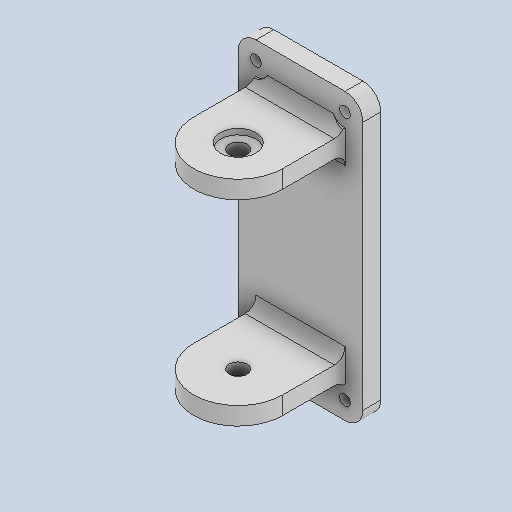
# Autodesk Inventor part: UnionBrazoPantalla
Saved by Autodesk Inventor 2023 (Build 270158000, 158)
## iProperties
Created: 2023-05-13
Part Number: UnionBrazoPantalla
Material: Genérico
Document SubType Name: Modeling
Designer: sergi
Density: 1 g/cm^3
Appearance: Valor por defecto
Author: sergi
Autodesk Inventor part; units mm, degrees
note: some values were not read from the file. Chosen so that the rebuilt part matches the saved one: direction of "Agujero1"; direction of "Agujero2".
ref_plane "YZ Plane" through (0, 0, 0) normal (1, 0, 0) x (0, 1, 0)
ref_plane "XZ Plane" through (0, 0, 0) normal (0, 1, 0) x (-1, 0, 0)
ref_plane "XY Plane" through (0, 0, 0) normal (0, 0, 1) x (1, 0, 0)
sketch "Boceto1" plane through (0, 0, 0) normal (0, 0, 1) x (1, 0, 0)
  line L0 (75.85, 9) -> (75.85, -9) projected
  line L1 (75.85, 9) -> (95.85, 9) projected
  line L2 (95.85, -9) -> (95.85, 9) projected
  line L3 (105.85, -146.9) -> (105.85, 146.9) projected
  line L4 (105.85, 146.9) -> (112.15, 146.9) projected
  line L5 (112.15, 146.9) -> (112.15, 160) projected
  line L6 (112.15, 160) -> (105.85, 160) projected
  line L7 (105.85, 160) -> (105.85, 180) projected
  line L8 (105.85, 180) -> (-100.9, 180) projected
  line L9 (-100.9, 180) -> (-100.9, 160) projected
  line L10 (-100.9, 160) -> (-108.4, 160) projected
  line L11 (-108.4, 160) -> (-108.4, 145) projected
  line L12 (-108.4, 145) -> (-100.9, 145) projected
  line L13 (-100.9, 145) -> (-100.9, 142) projected
  line L14 (-100.9, 142) -> (-112.15, 142) projected
  line L15 (-112.15, 142) -> (-112.15, -142) projected
  line L16 (15.85, 9) -> (15.85, -9) projected
  line L17 (15.85, 9) -> (35.85, 9) projected
  line L18 (35.85, -9) -> (35.85, 9) projected
  line L19 (20.45, 169.8) -> (20.45, 163.3) projected
  line L20 (20.45, 163.3) -> (13.95, 163.3) projected
  line L21 (13.95, 163.3) -> (13.95, 169.8) projected
  line L22 (13.95, 169.8) -> (20.45, 169.8) projected
  line L23 (78.15, 169.8) -> (78.15, 163.3) projected
  line L24 (78.15, 163.3) -> (71.65, 163.3) projected
  line L25 (71.65, 163.3) -> (71.65, 169.8) projected
  line L26 (71.65, 169.8) -> (78.15, 169.8) projected
  line L27 (-4.15, 163.3) -> (-4.15, 169.8) projected
  line L28 (-4.15, 169.8) -> (2.35, 169.8) projected
  line L29 (2.35, 169.8) -> (2.35, 163.3) projected
  line L30 (2.35, 163.3) -> (-4.15, 163.3) projected
  line L31 (38.55, 169.8) -> (38.55, 163.3) projected
  line L32 (38.55, 163.3) -> (32.05, 163.3) projected
  line L33 (32.05, 163.3) -> (32.05, 169.8) projected
  line L34 (32.05, 169.8) -> (38.55, 169.8) projected
  line L35 (56.65, 169.8) -> (56.65, 163.3) projected
  line L36 (56.65, 163.3) -> (50.15, 163.3) projected
  line L37 (50.15, 163.3) -> (50.15, 169.8) projected
  line L38 (50.15, 169.8) -> (56.65, 169.8) projected
  line L39 (-14.65, 175.8) -> (-14.65, 157.7) projected
  line L40 (-14.65, 157.7) -> (-22.65, 157.7) projected
  line L41 (-22.65, 157.7) -> (-22.65, 175.8) projected
  line L42 (-22.65, 175.8) -> (-14.65, 175.8) projected
  line L43 (35.85, -9) -> (35.85, 9) projected
  line L44 (35.85, -9) -> (15.85, -9) projected
  line L45 (15.85, 9) -> (15.85, -9) projected
  line L46 (-112.15, 142) -> (-112.15, -142) projected
  line L47 (-112.15, -142) -> (-100.9, -142) projected
  line L48 (-100.9, -142) -> (-100.9, -145) projected
  line L49 (-100.9, -145) -> (-108.4, -145) projected
  line L50 (-108.4, -145) -> (-108.4, -160) projected
  line L51 (-108.4, -160) -> (-100.9, -160) projected
  line L52 (-100.9, -160) -> (-100.9, -180) projected
  line L53 (-100.9, -180) -> (105.85, -180) projected
  line L54 (105.85, -180) -> (105.85, -160) projected
  line L55 (105.85, -160) -> (112.15, -160) projected
  line L56 (112.15, -160) -> (112.15, -146.9) projected
  line L57 (112.15, -146.9) -> (105.85, -146.9) projected
  line L58 (105.85, -146.9) -> (105.85, 146.9) projected
  line L59 (95.85, -9) -> (95.85, 9) projected
  line L60 (95.85, -9) -> (75.85, -9) projected
  line L61 (75.85, 9) -> (75.85, -9) projected
  circle A0 centre (-103.8, -156.7) radius 1.5 projected
  line L62 (-25.85, -52.4) -> (-25.85, -57.4) projected
  line L63 (-25.85, -57.4) -> (-8.15, -57.4) projected
  arc A1 (-3.15, -62.4) -> (-8.15, -57.4) centre (-8.15, -62.4) ccw projected
  line L64 (-3.15, -62.4) -> (-3.15, -87.4) projected
  line L65 (-3.15, -87.4) -> (-2.05, -87.4) projected
  line L66 (-2.05, -87.4) -> (-2.05, -107.4) projected
  line L67 (-2.05, -107.4) -> (-3.15, -107.4) projected
  line L68 (-3.15, -107.4) -> (-3.15, -169.7804) projected
  arc A2 (-8.15, -174.7804) -> (-3.15, -169.7804) centre (-8.15, -169.7804) ccw projected
  line L69 (-8.15, -174.7804) -> (-67.5256, -174.7804) projected
  line L70 (-67.5256, -174.7804) -> (-67.5256, -57.4) projected
  line L71 (-67.5256, -57.4) -> (-48.05, -57.4) projected
  line L72 (-48.05, -57.4) -> (-48.05, -52.4) projected
  line L73 (-48.05, -52.4) -> (-25.85, -52.4) projected
  line L74 (-112.15, 0) -> (-67.15, 0)
  line L75 (-67.15, 0) -> (-67.15, -40)
  line L76 (-67.15, -40) -> (-32.15, -40)
  line L77 (-32.15, -40) -> (-32.15, 40)
  line L78 (-32.15, 40) -> (-67.15, 40)
  line L79 (-67.15, 40) -> (-67.15, 0)
  line L80 (-37.15, 35) -> (-37.15, -35)
  line L81 (-37.15, -35) -> (-62.15, -35)
  line L82 (-62.15, -35) -> (-62.15, 0)
  line L83 (-62.15, 0) -> (-62.15, 35)
  line L84 (-62.15, 35) -> (-37.15, 35)
  circle A3 centre (-37.15, 35) radius 1.5
  circle A4 centre (-37.15, -35) radius 1.5
  circle A5 centre (-62.15, -35) radius 1.5
  circle A6 centre (-62.15, 35) radius 1.5
  circle A7 centre (-37.15, -35) radius 1.6 projected
  circle A8 centre (-37.15, 35) radius 1.6 projected
  circle A9 centre (-62.15, 35) radius 1.6 projected
  circle A10 centre (-62.15, -35) radius 1.6 projected
  line L85 (75.85, 9) -> (95.85, 9) projected
  line L86 (15.85, 9) -> (35.85, 9) projected
  line L87 (20.45, 169.8) -> (20.45, 163.3) projected
  line L88 (20.45, 163.3) -> (13.95, 163.3) projected
  line L89 (13.95, 163.3) -> (13.95, 169.8) projected
  line L90 (13.95, 169.8) -> (20.45, 169.8) projected
  line L91 (78.15, 169.8) -> (78.15, 163.3) projected
  line L92 (78.15, 163.3) -> (71.65, 163.3) projected
  line L93 (71.65, 163.3) -> (71.65, 169.8) projected
  line L94 (71.65, 169.8) -> (78.15, 169.8) projected
  line L95 (-4.15, 163.3) -> (-4.15, 169.8) projected
  line L96 (-4.15, 169.8) -> (2.35, 169.8) projected
  line L97 (2.35, 169.8) -> (2.35, 163.3) projected
  line L98 (2.35, 163.3) -> (-4.15, 163.3) projected
  line L99 (38.55, 169.8) -> (38.55, 163.3) projected
  line L100 (38.55, 163.3) -> (32.05, 163.3) projected
  line L101 (32.05, 163.3) -> (32.05, 169.8) projected
  line L102 (32.05, 169.8) -> (38.55, 169.8) projected
  line L103 (56.65, 169.8) -> (56.65, 163.3) projected
  line L104 (56.65, 163.3) -> (50.15, 163.3) projected
  line L105 (50.15, 163.3) -> (50.15, 169.8) projected
  line L106 (50.15, 169.8) -> (56.65, 169.8) projected
  line L107 (-14.65, 175.8) -> (-14.65, 157.7) projected
  line L108 (-14.65, 157.7) -> (-22.65, 157.7) projected
  line L109 (-22.65, 157.7) -> (-22.65, 175.8) projected
  line L110 (-22.65, 175.8) -> (-14.65, 175.8) projected
  line L111 (-100.9, 142) -> (-112.15, 142) projected
  line L112 (105.85, 146.9) -> (112.15, 146.9) projected
  line L113 (112.15, 146.9) -> (112.15, 160) projected
  line L114 (112.15, 160) -> (105.85, 160) projected
  line L115 (105.85, 160) -> (105.85, 180) projected
  line L116 (105.85, 180) -> (-100.9, 180) projected
  line L117 (-100.9, 180) -> (-100.9, 160) projected
  line L118 (-100.9, 160) -> (-108.4, 160) projected
  line L119 (-108.4, 160) -> (-108.4, 145) projected
  line L120 (-108.4, 145) -> (-100.9, 145) projected
  line L121 (-100.9, 145) -> (-100.9, 142) projected
  circle A11 centre (-37.15, -35) radius 1.6 projected
  circle A12 centre (-37.15, 35) radius 1.6 projected
  circle A13 centre (-62.15, 35) radius 1.6 projected
  circle A14 centre (-62.15, -35) radius 1.6 projected
  line L122 (95.85, -9) -> (75.85, -9) projected
  line L123 (35.85, -9) -> (15.85, -9) projected
  line L124 (-25.85, -52.4) -> (-25.85, -57.4) projected
  line L125 (-25.85, -57.4) -> (-8.15, -57.4) projected
  arc A15 (-3.15, -62.4) -> (-8.15, -57.4) centre (-8.15, -62.4) ccw projected
  line L126 (-3.15, -62.4) -> (-3.15, -87.4) projected
  line L127 (-3.15, -87.4) -> (-2.05, -87.4) projected
  line L128 (-2.05, -87.4) -> (-2.05, -107.4) projected
  line L129 (-2.05, -107.4) -> (-3.15, -107.4) projected
  line L130 (-3.15, -107.4) -> (-3.15, -169.7804) projected
  arc A16 (-8.15, -174.7804) -> (-3.15, -169.7804) centre (-8.15, -169.7804) ccw projected
  line L131 (-8.15, -174.7804) -> (-67.5256, -174.7804) projected
  line L132 (-67.5256, -174.7804) -> (-67.5256, -57.4) projected
  line L133 (-67.5256, -57.4) -> (-48.05, -57.4) projected
  line L134 (-48.05, -57.4) -> (-48.05, -52.4) projected
  line L135 (-48.05, -52.4) -> (-25.85, -52.4) projected
  circle A17 centre (-103.8, -156.7) radius 1.5 projected
  line L136 (-112.15, -142) -> (-100.9, -142) projected
  line L137 (-100.9, -142) -> (-100.9, -145) projected
  line L138 (-100.9, -145) -> (-108.4, -145) projected
  line L139 (-108.4, -145) -> (-108.4, -160) projected
  line L140 (-108.4, -160) -> (-100.9, -160) projected
  line L141 (-100.9, -160) -> (-100.9, -180) projected
  line L142 (-100.9, -180) -> (105.85, -180) projected
  line L143 (105.85, -180) -> (105.85, -160) projected
  line L144 (105.85, -160) -> (112.15, -160) projected
  line L145 (112.15, -160) -> (112.15, -146.9) projected
  line L146 (112.15, -146.9) -> (105.85, -146.9) projected
  dimension "d0" = 45
  dimension "d1" = 40
  dimension "d2" = 35
  dimension "d3" = 80
  dimension "d4" = 5
  dimension "d5" = 3
  dimension "d6" = 3
  dimension "d7" = 3
  dimension "d8" = 3
  constraints: 22 end point, 8 perpendicular, 4 centre point, 4 coincident, 1 point on line, 4 other
  measures "d0" distance of L74.start L74.end
  measures "d1" distance of L74.end L75.end
  measures "d2" distance of L75.end L76.end
  measures "d3" distance of L76.end L77.end
  measures "d4" distance between parallel lines of L77 L80
  measures "d5" diameter of A3
  measures "d6" diameter of A4
  measures "d7" diameter of A5
  measures "d8" diameter of A6
extrude "Extrusión1" add sketch "Boceto1" along normal blind 5 contours L79 L78 L77 L76 L75 | A3 L84 A8 L80 | L80 A8 L84 A3 | L80 A7 L81 A10 L82 L83 A9 L84 A8 | A7 L81 A4 L80 | L80 A4 L81 A7 | A9 L83 A6 L84 | L84 A6 L83 A9 | A10 L82 A5 L81 | L81 A5 L82 A10
sketch "Boceto2" plane through (0, 0, 5) normal (0, 0, 1) x (1, 0, 0)
  circle A0 centre (-37.15, 35) radius 1.5 projected
  circle A1 centre (-62.15, -35) radius 1.5 projected
  line L0 (-37.15, 35) -> (-62.15, 35)
  line L1 (-62.15, 35) -> (-62.15, -35)
  line L2 (-62.15, -35) -> (-37.15, -35)
  line L3 (-37.15, -35) -> (-37.15, 35)
  line L4 (-50.6099, 35) -> (-50.6099, 30)
  line L5 (-37.15, 30) -> (-62.15, 30)
  line L6 (-37.15, 25) -> (-62.15, 25)
  line L7 (-49.65, -35) -> (-49.65, -30)
  line L8 (-49.65, -25) -> (-37.15, -25)
  line L9 (-49.65, -30) -> (-37.15, -30)
  line L10 (-49.65, -30) -> (-62.15, -30)
  line L11 (-62.15, -30) -> (-37.15, -30)
  line L12 (-37.15, -30) -> (-37.15, -25)
  line L13 (-37.15, -25) -> (-62.15, -25)
  line L14 (-62.15, -25) -> (-62.15, -30)
  point P0 (0, 0)
  dimension "d11" = 5
  dimension "d12" = 5
  dimension "d13" = 5
  dimension "d14" = 5
  constraints: 30 end point, 8 point on line, 6 parallel, 4 perpendicular, 3 horizontal, 1 midpoint, 1 vertical
  measures "d11" distance of L4.start L4.end
  measures "d12" distance between parallel lines of L5 L6
  measures "d13" distance of L7.start L7.end
  measures "d14" distance of L7.end L8.start
extrude "Extrusión2" add sketch "Boceto2" along normal blind 30 contours L3 L6 L1 L5 | L3 L9 L10 L1 L13 L8
fillet "Empalme1" radius 12.5 4 edges at (-37.15, 27.5, 35) (-62.15, 27.5, 35) (-37.15, -27.5, 35) (-62.15, -27.5, 35)
fillet "Empalme2" radius 3 4 edges at (-49.65, 30, 5) (-49.65, 25, 5) (-49.65, -25, 5) (-49.65, -30, 5)
sketch "Boceto3" plane through (0, 0, 5) normal (0, 0, 1) x (1, 0, 0)
  line L0 (-62.15, -33) -> (-62.15, -22) projected
  line L1 (-37.15, -22) -> (-62.15, -22) projected
  line L2 (-37.15, -22) -> (-37.15, -33) projected
  line L3 (-62.15, -33) -> (-37.15, -33) projected
  line L4 (-62.15, 22) -> (-62.15, 33) projected
  line L5 (-37.15, 33) -> (-62.15, 33) projected
  line L6 (-37.15, 33) -> (-37.15, 22) projected
  line L7 (-62.15, 22) -> (-37.15, 22) projected
  line L8 (-32.15, 40) -> (-67.15, 40) projected
  line L9 (-67.15, 40) -> (-67.15, -40) projected
  line L10 (-67.15, -40) -> (-32.15, -40) projected
  line L11 (-32.15, -40) -> (-32.15, 40) projected
  circle A0 centre (-62.15, -35) radius 1.5 projected
  circle A1 centre (-37.15, -35) radius 1.5 projected
  circle A2 centre (-37.15, 35) radius 1.5 projected
  circle A3 centre (-62.15, 35) radius 1.5 projected
  circle A4 centre (-62.15, 35) radius 3.9
  circle A5 centre (-37.15, 35) radius 3.9
  circle A6 centre (-62.15, -35) radius 1.5 projected
  circle A7 centre (-62.15, -35) radius 3.9
  circle A8 centre (-37.15, -35) radius 3.9
  point P0 (0, 0)
  dimension "d19" = 7.8
  dimension "d20" = 7.8
  dimension "d21" = 7.8
  dimension "d22" = 7.8
  constraints: 4 centre point, 4 coincident
  measures "d19" diameter of A4
  measures "d20" diameter of A5
  measures "d21" diameter of A7
  measures "d22" diameter of A8
extrude "Extrusión3" cut sketch "Boceto3" along normal blind 30 contours L3 A7 L0 | L0 A7 L3 | A8 L2 L3 | L3 L2 A8 | A4 L5 L4 | L4 L5 A4 | A5 L5 L6 | L6 L5 A5
sketch "Boceto4" plane through (-49.65, 30, 22.5) normal (0, 1, 0) x (1, 0, 0)
  arc A0 (-12.5, 0) -> (12.5, 0) centre (0, 0) ccw projected
  point P0 (49.65, 22.5)
  constraints: 1 coincident
hole "Agujero1" at (-49.65, 30, 22.5) direction (0, -1, 0) diameter 5 depth 5 counterbore diameter 10 counterbore depth 1.6
sketch "Boceto5" plane through (-49.65, -30, 22.5) normal (0, -1, 0) x (1, 0, 0)
  arc A0 (12.5, 0) -> (-12.5, 0) centre (0, 0) ccw projected
  point P0 (49.65, -22.5)
  constraints: 2 coincident
hole "Agujero2" at (-49.65, -30, 22.5) direction (0, 1, 0) diameter 5 depth 5 counterbore diameter 10 counterbore depth 1.6
fillet "Empalme3" radius 5 4 edges at (-32.15, 40, 2.5) (-67.15, 40, 2.5) (-67.15, -40, 2.5) (-32.15, -40, 2.5)
